Hedgehog (Autodesk Fusion 360 design; units mm, degrees)
Autodesk Fusion 360 part; units mm, degrees
note: some values were not read from the file. Set by a fixed rule: which sketch regions a step uses.
(part 1 of 2)
sketch "Sketch4" plane through (0, 0, 0) normal (0, 0, 1) x (1, 0, 0)
  line L0 (-34.7307, 191.5789) -> (1016.2208, 191.5789)
  line L1 (1016.2208, 191.5789) -> (1016.2208, -23.2363)
  line L2 (1016.2208, -23.2363) -> (-34.7307, -23.2363)
  line L3 (-34.7307, -23.2363) -> (-34.7307, 191.5789)
  line L4 (-14.0403, 161.1518) -> (163.6539, 161.1518)
  line L5 (163.6539, 161.1518) -> (163.6539, 10.2335)
  line L6 (163.6539, 10.2335) -> (-14.0403, 10.2335)
  line L7 (-14.0403, 10.2335) -> (-14.0403, 161.1518)
  spline S0 degree 3 poles (109.5886, 49.3104) (109.6257, 48.0501) (109.3099, 46.9639) (108.2091, 46.2939) knots 0 0 0 0 1 1 1 1
  spline S1 degree 3 poles (108.2091, 46.2939) (107.8993, 46.1052) (107.561, 45.9726) (107.2226, 45.8399) knots 0 0 0 0 1 1 1 1
  spline S2 degree 3 poles (107.2226, 45.8399) (106.9189, 45.7212) (106.6147, 45.602) (106.3317, 45.4419) knots 0 0 0 0 1 1 1 1
  spline S3 degree 3 poles (106.3317, 45.4419) (105.6678, 45.067) (105.1207, 44.4463) (104.9491, 43.7039) knots 0 0 0 0 1 1 1 1
  spline S4 degree 3 poles (104.9491, 43.7039) (104.7763, 42.9615) (105.0288, 42.1089) (105.6477, 41.6641) knots 0 0 0 0 1 1 1 1
  spline S5 degree 3 poles (105.6477, 41.6641) (106.1254, 41.3209) (106.7419, 41.2497) (107.3297, 41.215) knots 0 0 0 0 1 1 1 1
  spline S6 degree 3 poles (107.3297, 41.215) (111.923, 40.9454) (115.0552, 41.6239) (115.8079, 46.7503) knots 0 0 0 0 1 1 1 1
  spline S7 degree 3 poles (115.8079, 46.7503) (115.9868, 47.9716) (116.1183, 49.2307) (116.1183, 50.4764) knots 0 0 0 0 1 1 1 1
  spline S8 degree 3 poles (116.1183, 50.4764) (119.4056, 51.2164) (122.0869, 52.1176) (123.8121, 53.1838) knots 0 0 0 0 1 1 1 1
  spline S9 degree 3 poles (123.8121, 53.1838) (124.4796, 53.5958) (125.3535, 53.8209) (126.189, 54.0357) knots 0 0 0 0 1 1 1 1
  spline S10 degree 3 poles (126.189, 54.0357) (127.9082, 54.4781) (129.4685, 54.8798) (128.7577, 56.787) knots 0 0 0 0 1 1 1 1
  line L8 (128.7577, 56.787) -> (128.6384, 57.1442)
  spline S11 degree 3 poles (128.6384, 57.1442) (129.9656, 57.2215) (132.1333, 57.3943) (133.0443, 57.7314) knots 0 0 0 0 1 1 1 1
  spline S12 degree 2 poles (133.0443, 57.7314) (134.4098, 58.2371) (132.3493, 63.2089) knots 0 0 0 1 1 1
  spline S13 degree 2 poles (132.3493, 63.2089) (136.6432, 62.0015) (138.6368, 64.3663) knots 0 0 0 1 1 1
  spline S14 degree 2 poles (138.6368, 64.3663) (140.6522, 66.7567) (129.92, 74.047) knots 0 0 0 1 1 1
  spline S15 degree 2 poles (129.92, 74.047) (135.9093, 73.8967) (138.2637, 76.3917) knots 0 0 0 1 1 1
  spline S16 degree 2 poles (138.2637, 76.3917) (140.6474, 78.9184) (126.1945, 83.6042) knots 0 0 0 1 1 1
  spline S17 degree 2 poles (126.1945, 83.6042) (133.7788, 85.2917) (134.9922, 88.733) knots 0 0 0 1 1 1
  spline S18 degree 2 poles (134.9922, 88.733) (136.216, 92.2041) (121.0608, 94.2177) knots 0 0 0 1 1 1
  spline S19 degree 2 poles (121.0608, 94.2177) (130.8541, 97.9883) (130.6527, 101.1843) knots 0 0 0 1 1 1
  spline S20 degree 2 poles (130.6527, 101.1843) (130.4506, 104.3889) (113.1942, 101.9815) knots 0 0 0 1 1 1
  spline S21 degree 2 poles (113.1942, 101.9815) (122.5828, 107.2837) (121.0475, 109.7769) knots 0 0 0 1 1 1
  spline S22 degree 2 poles (121.0475, 109.7769) (119.5182, 112.2598) (100.8633, 108.6761) knots 0 0 0 1 1 1
  spline S23 degree 2 poles (100.8633, 108.6761) (113.2813, 116.3687) (110.9798, 119.6566) knots 0 0 0 1 1 1
  spline S24 degree 2 poles (110.9798, 119.6566) (107.9042, 124.0497) (89.2098, 113.5389) knots 0 0 0 1 1 1
  spline S25 degree 2 poles (89.2098, 113.5389) (99.8374, 122.5539) (97.3934, 126.0025) knots 0 0 0 1 1 1
  spline S26 degree 2 poles (97.3934, 126.0025) (94.9672, 129.4249) (77.9353, 116.7569) knots 0 0 0 1 1 1
  spline S27 degree 2 poles (77.9353, 116.7569) (83.1292, 123.5397) (81.9913, 126.8745) knots 0 0 0 1 1 1
  spline S28 degree 2 poles (81.9913, 126.8745) (80.8563, 130.2032) (63.1064, 114.8084) knots 0 0 0 1 1 1
  spline S29 degree 2 poles (63.1064, 114.8084) (68.0374, 122.6482) (66.5075, 124.7586) knots 0 0 0 1 1 1
  spline S30 degree 3 poles (66.5075, 124.7586) (65.3872, 126.3043) (56.8159, 118.2697) (51.9068, 113.6679) knots 0 0 0 0 1 1 1 1
  spline S31 degree 3 poles (51.9068, 113.6679) (50.1475, 112.0188) (48.8586, 110.8102) (48.5519, 110.6423) knots 0 0 0 0 1 1 1 1
  spline S32 degree 3 poles (48.5519, 110.6423) (48.1119, 110.4007) (48.3407, 111.3738) (48.6724, 112.788) knots 0 0 0 0 1 1 1 1
  spline S33 degree 3 poles (48.6724, 112.788) (49.2122, 115.0877) (50.0252, 118.5527) (48.6839, 119.8562) knots 0 0 0 0 1 1 1 1
  spline S34 degree 3 poles (48.6839, 119.8562) (46.9715, 121.5206) (41.6425, 110.8108) (38.6625, 104.821) knots 0 0 0 0 1 1 1 1
  spline S35 degree 3 poles (38.6625, 104.821) (37.9055, 103.2996) (37.3, 102.0831) (36.944, 101.4509) knots 0 0 0 0 1 1 1 1
  spline S36 degree 3 poles (36.944, 101.4509) (36.0518, 99.8662) (35.537, 101.7697) (34.8987, 104.1303) knots 0 0 0 0 1 1 1 1
  spline S37 degree 3 poles (34.8987, 104.1303) (34.2944, 106.3642) (33.5793, 109.0077) (32.3294, 109.494) knots 0 0 0 0 1 1 1 1
  spline S38 degree 3 poles (32.3294, 109.494) (29.7893, 110.4822) (30.3547, 93.6694) (30.6571, 90.6164) knots 0 0 0 0 1 1 1 1
  spline S39 degree 3 poles (30.6571, 90.6164) (30.8026, 89.1468) (29.053, 90.2245) (27.318, 91.2931) knots 0 0 0 0 1 1 1 1
  spline S40 degree 3 poles (27.318, 91.2931) (25.4549, 92.4402) (23.6081, 93.5776) (24.1413, 91.5414) knots 0 0 0 0 1 1 1 1
  spline S41 degree 2 poles (24.1413, 91.5414) (25.1718, 87.6041) (28.5546, 81.4019) knots 0 0 0 1 1 1
  spline S42 degree 2 poles (28.5546, 81.4019) (22.02, 79.7004) (25.3388, 77.663) knots 0 0 0 1 1 1
  spline S43 degree 3 poles (25.3388, 77.663) (27.4805, 76.3479) (29.9591, 72.7204) (31.4829, 70.2485) knots 0 0 0 0 1 1 1 1
  spline S44 degree 3 poles (31.4829, 70.2485) (24.6857, 66.904) (19.2909, 63.9525) (22.1953, 61.5847) knots 0 0 0 0 1 1 1 1
  spline S45 degree 3 poles (22.1953, 61.5847) (24.3014, 59.8674) (32.417, 58.4872) (39.0288, 57.3626) knots 0 0 0 0 1 1 1 1
  spline S46 degree 3 poles (39.0288, 57.3626) (41.7143, 56.9056) (44.1515, 56.4912) (45.8378, 56.1133) knots 0 0 0 0 1 1 1 1
  spline S47 degree 3 poles (45.8378, 56.1133) (47.005, 55.8522) (48.1685, 55.5248) (49.374, 55.1475) knots 0 0 0 0 1 1 1 1
  line L9 (49.374, 55.1475) -> (49.3771, 55.1342)
  spline S48 degree 3 poles (49.3771, 55.1342) (49.9089, 52.5886) (50.4609, 49.9488) (48.4138, 48.7718) knots 0 0 0 0 1 1 1 1
  spline S49 degree 3 poles (48.4138, 48.7718) (48.0998, 48.5911) (47.7584, 48.4676) (47.417, 48.3441) knots 0 0 0 0 1 1 1 1
  spline S50 degree 3 poles (47.417, 48.3441) (47.1096, 48.2321) (46.8023, 48.1207) (46.5145, 47.968) knots 0 0 0 0 1 1 1 1
  spline S51 degree 3 poles (46.5145, 47.968) (45.8421, 47.6101) (45.2792, 47.0034) (45.0887, 46.2659) knots 0 0 0 0 1 1 1 1
  spline S52 degree 3 poles (45.0887, 46.2659) (44.897, 45.5283) (45.1288, 44.6691) (45.7356, 44.209) knots 0 0 0 0 1 1 1 1
  spline S53 degree 3 poles (45.7356, 44.209) (46.2047, 43.8536) (46.8194, 43.7666) (47.406, 43.7173) knots 0 0 0 0 1 1 1 1
  spline S54 degree 3 poles (47.406, 43.7173) (51.9902, 43.3315) (55.1387, 43.9297) (56.0205, 49.036) knots 0 0 0 0 1 1 1 1
  spline S55 degree 3 poles (56.0205, 49.036) (56.2317, 50.2549) (56.3948, 51.5133) (56.4264, 52.7602) knots 0 0 0 0 1 1 1 1
  spline S56 degree 3 poles (56.4264, 52.7602) (57.8011, 52.2965) (59.2805, 51.814) (60.9004, 51.3241) knots 0 0 0 0 1 1 1 1
  spline S57 degree 3 poles (60.9004, 51.3241) (61.2741, 49.2471) (61.3453, 47.2943) (59.6645, 46.3279) knots 0 0 0 0 1 1 1 1
  spline S58 degree 3 poles (59.6645, 46.3279) (59.3505, 46.1478) (59.0097, 46.0243) (58.6683, 45.9001) knots 0 0 0 0 1 1 1 1
  spline S59 degree 3 poles (58.6683, 45.9001) (58.361, 45.7888) (58.0537, 45.6774) (57.7652, 45.5241) knots 0 0 0 0 1 1 1 1
  spline S60 degree 3 poles (57.7652, 45.5241) (57.0928, 45.1668) (56.5311, 44.5595) (56.3394, 43.822) knots 0 0 0 0 1 1 1 1
  spline S61 degree 3 poles (56.3394, 43.822) (56.1483, 43.0844) (56.379, 42.2258) (56.9863, 41.7657) knots 0 0 0 0 1 1 1 1
  spline S62 degree 3 poles (56.9863, 41.7657) (57.4549, 41.4097) (58.0701, 41.3227) (58.6567, 41.2734) knots 0 0 0 0 1 1 1 1
  spline S63 degree 3 poles (58.6567, 41.2734) (63.2415, 40.8876) (66.3895, 41.4864) (67.2719, 46.5921) knots 0 0 0 0 1 1 1 1
  spline S64 degree 3 poles (67.2719, 46.5921) (67.4368, 47.5432) (67.5719, 48.5187) (67.6382, 49.4942) knots 0 0 0 0 1 1 1 1
  spline S65 degree 3 poles (67.6382, 49.4942) (68.0222, 49.4011) (68.4129, 49.3086) (68.8109, 49.2167) knots 0 0 0 0 1 1 1 1
  spline S66 degree 3 poles (68.8109, 49.2167) (74.0942, 47.9929) (84.3688, 47.5682) (94.7646, 48.0142) knots 0 0 0 0 1 1 1 1
  spline S67 degree 3 poles (94.7646, 48.0142) (94.5473, 47.5968) (94.2205, 47.2359) (93.7519, 46.9505) knots 0 0 0 0 1 1 1 1
  spline S68 degree 3 poles (93.7519, 46.9505) (93.4422, 46.7624) (93.1044, 46.6298) (92.7667, 46.4977) knots 0 0 0 0 1 1 1 1
  spline S69 degree 3 poles (92.7667, 46.4977) (92.4624, 46.3785) (92.1576, 46.2592) (91.8734, 46.0985) knots 0 0 0 0 1 1 1 1
  spline S70 degree 3 poles (91.8734, 46.0985) (91.2101, 45.7243) (90.6636, 45.103) (90.492, 44.3605) knots 0 0 0 0 1 1 1 1
  spline S71 degree 3 poles (90.492, 44.3605) (90.3192, 43.6187) (90.5711, 42.7655) (91.1906, 42.3207) knots 0 0 0 0 1 1 1 1
  spline S72 degree 3 poles (91.1906, 42.3207) (91.6683, 41.9775) (92.2847, 41.9063) (92.872, 41.8722) knots 0 0 0 0 1 1 1 1
  spline S73 degree 3 poles (92.872, 41.8722) (97.4659, 41.602) (100.5968, 42.2799) (101.3496, 47.4063) knots 0 0 0 0 1 1 1 1
  spline S74 degree 3 poles (101.3496, 47.4063) (101.3995, 47.744) (101.4451, 48.0848) (101.4859, 48.4274) knots 0 0 0 0 1 1 1 1
  spline S75 degree 3 poles (101.4859, 48.4274) (104.2907, 48.6544) (107.0254, 48.9483) (109.5886, 49.3104) knots 0 0 0 0 1 1 1 1
  line L10 (193.4724, 161.1518) -> (371.1666, 161.1518)
  line L11 (371.1666, 161.1518) -> (371.1666, 10.2335)
  line L12 (371.1666, 10.2335) -> (193.4724, 10.2335)
  line L13 (193.4724, 10.2335) -> (193.4724, 161.1518)
  spline S76 degree 3 poles (261.6784, 59.7712) (261.0309, 60.2988) (260.2082, 60.5623) (259.3878, 60.7175) knots 0 0 0 0 1 1 1 1
  spline S77 degree 3 poles (259.3878, 60.7175) (257.7259, 61.0315) (256.9239, 60.5118) (256.5977, 59.5576) knots 0 0 0 0 1 1 1 1
  spline S78 degree 3 poles (256.5977, 59.5576) (255.6009, 56.6464) (259.3069, 50.7143) (255.9265, 48.7718) knots 0 0 0 0 1 1 1 1
  spline S79 degree 3 poles (255.9265, 48.7718) (255.3295, 48.4286) (254.6351, 48.2911) (254.0272, 47.968) knots 0 0 0 0 1 1 1 1
  spline S80 degree 3 poles (254.0272, 47.968) (253.3548, 47.6101) (252.7919, 47.0034) (252.6014, 46.2659) knots 0 0 0 0 1 1 1 1
  spline S81 degree 3 poles (252.6014, 46.2659) (252.4097, 45.5283) (252.6415, 44.6691) (253.2483, 44.209) knots 0 0 0 0 1 1 1 1
  spline S82 degree 3 poles (253.2483, 44.209) (253.7175, 43.8536) (254.3321, 43.7666) (254.9187, 43.7173) knots 0 0 0 0 1 1 1 1
  spline S83 degree 3 poles (254.9187, 43.7173) (259.5035, 43.3315) (262.6515, 43.9297) (263.5332, 49.036) knots 0 0 0 0 1 1 1 1
  spline S84 degree 3 poles (263.5332, 49.036) (264.0688, 52.1304) (264.297, 55.4768) (262.8413, 58.2596) knots 0 0 0 0 1 1 1 1
  spline S85 degree 3 poles (262.8413, 58.2596) (262.5444, 58.8268) (262.175, 59.3672) (261.6784, 59.7712) knots 0 0 0 0 1 1 1 1
  spline S86 degree 3 poles (306.736, 58.0917) (306.0764, 58.6022) (305.2463, 58.8456) (304.4224, 58.9795) knots 0 0 0 0 1 1 1 1
  spline S87 degree 3 poles (304.4224, 58.9795) (302.7544, 59.2509) (301.9651, 58.7124) (301.662, 57.7491) knots 0 0 0 0 1 1 1 1
  spline S88 degree 3 poles (301.662, 57.7491) (300.7407, 54.8147) (304.5952, 48.9781) (301.2647, 46.9505) knots 0 0 0 0 1 1 1 1
  spline S89 degree 3 poles (301.2647, 46.9505) (300.6762, 46.5927) (299.9861, 46.4369) (299.3861, 46.0985) knots 0 0 0 0 1 1 1 1
  spline S90 degree 3 poles (299.3861, 46.0985) (298.7228, 45.7243) (298.1763, 45.103) (298.0047, 44.3605) knots 0 0 0 0 1 1 1 1
  spline S91 degree 3 poles (298.0047, 44.3605) (297.8319, 43.6187) (298.0838, 42.7655) (298.7033, 42.3207) knots 0 0 0 0 1 1 1 1
  spline S92 degree 3 poles (298.7033, 42.3207) (299.181, 41.9775) (299.7975, 41.9063) (300.3853, 41.8722) knots 0 0 0 0 1 1 1 1
  spline S93 degree 3 poles (300.3853, 41.8722) (304.9786, 41.602) (308.1095, 42.2799) (308.8623, 47.4063) knots 0 0 0 0 1 1 1 1
  spline S94 degree 3 poles (308.8623, 47.4063) (309.3193, 50.5141) (309.4629, 53.8641) (307.9367, 56.6099) knots 0 0 0 0 1 1 1 1
  spline S95 degree 3 poles (307.9367, 56.6099) (307.6257, 57.1691) (307.243, 57.7004) (306.736, 58.0917) knots 0 0 0 0 1 1 1 1
  line L14 (335.9661, 57.6998) -> (335.3576, 58.3083)
  spline S96 degree 2 poles (335.3576, 58.3083) (334.174, 58.4331) (333.5362, 58.8603) knots 0 0 0 1 1 1
  spline S97 degree 3 poles (333.5362, 58.8603) (332.8972, 59.2868) (332.271, 59.7901) (331.5152, 59.9252) knots 0 0 0 0 1 1 1 1
  spline S98 degree 3 poles (331.5152, 59.9252) (331.6211, 58.7678) (331.8493, 57.6213) (332.1956, 56.5101) knots 0 0 0 0 1 1 1 1
  spline S99 degree 3 poles (332.1956, 56.5101) (329.9391, 56.6938) (328.1494, 58.4306) (326.6725, 60.1467) knots 0 0 0 0 1 1 1 1
  spline S100 degree 3 poles (326.6725, 60.1467) (326.1789, 60.7206) (325.5966, 61.4441) (324.8493, 61.4539) knots 0 0 0 0 1 1 1 1
  spline S101 degree 3 poles (324.8493, 61.4539) (324.7878, 60.9536) (327.6151, 55.4159) (326.4552, 55.6752) knots 0 0 0 0 1 1 1 1
  spline S102 degree 2 poles (326.4552, 55.6752) (324.7866, 56.0488) (313.0271, 62.1853) knots 0 0 0 1 1 1
  spline S103 degree 2 poles (313.0271, 62.1853) (315.7571, 54.0437) (313.4969, 54.8999) knots 0 0 0 1 1 1
  spline S104 degree 2 poles (313.4969, 54.8999) (311.2368, 55.7567) (302.27, 63.8071) knots 0 0 0 1 1 1
  spline S105 degree 2 poles (302.27, 63.8071) (301.9608, 56.1711) (300.238, 57.0815) knots 0 0 0 1 1 1
  spline S106 degree 2 poles (300.238, 57.0815) (298.5159, 57.9925) (289.95, 67.4419) knots 0 0 0 1 1 1
  spline S107 degree 2 poles (289.95, 67.4419) (289.2392, 58.4075) (286.3603, 60.0153) knots 0 0 0 1 1 1
  spline S108 degree 2 poles (286.3603, 60.0153) (283.4806, 61.6236) (276.9004, 72.9042) knots 0 0 0 1 1 1
  spline S109 degree 2 poles (276.9004, 72.9042) (282.7412, 84.9058) (273.8699, 84.0034) knots 0 0 0 1 1 1
  spline S110 degree 3 poles (273.8699, 84.0034) (269.7592, 83.5847) (266.3277, 82.0366) (264.4211, 78.1614) knots 0 0 0 0 1 1 1 1
  spline S111 degree 3 poles (264.4211, 78.1614) (262.9338, 79.7558) (260.6427, 80.4464) (258.4671, 80.3083) knots 0 0 0 0 1 1 1 1
  spline S112 degree 3 poles (258.4671, 80.3083) (256.4151, 80.099) (255.0283, 79.547) (253.1631, 78.6391) knots 0 0 0 0 1 1 1 1
  spline S113 degree 3 poles (253.1631, 78.6391) (252.7274, 78.4273) (252.2204, 78.2125) (251.7774, 78.4078) knots 0 0 0 0 1 1 1 1
  spline S114 degree 3 poles (251.7774, 78.4078) (251.4865, 78.5356) (251.2961, 78.8119) (251.0959, 79.0578) knots 0 0 0 0 1 1 1 1
  spline S115 degree 3 poles (251.0959, 79.0578) (250.3413, 79.987) (249.2343, 80.64) (248.0458, 80.7781) knots 0 0 0 0 1 1 1 1
  spline S116 degree 3 poles (248.0458, 80.7781) (246.8446, 80.9175) (244.5838, 80.3253) (244.2108, 78.9379) knots 0 0 0 0 1 1 1 1
  spline S117 degree 3 poles (244.2108, 78.9379) (244.6575, 80.5998) (245.3025, 82.9658) (244.5966, 84.6551) knots 0 0 0 0 1 1 1 1
  spline S118 degree 3 poles (244.5966, 84.6551) (244.4676, 84.9643) (244.2498, 85.2375) (243.979, 85.459) knots 0 0 0 0 1 1 1 1
  spline S119 degree 3 poles (243.979, 85.459) (243.1246, 86.16) (241.7407, 86.3505) (240.9442, 85.5472) knots 0 0 0 0 1 1 1 1
  spline S120 degree 3 poles (240.9442, 85.5472) (240.3161, 84.9138) (240.2875, 83.8768) (240.5839, 83.0352) knots 0 0 0 0 1 1 1 1
  spline S121 degree 3 poles (240.5839, 83.0352) (240.8803, 82.1942) (241.442, 81.4773) (241.8972, 80.7099) knots 0 0 0 0 1 1 1 1
  spline S122 degree 3 poles (241.8972, 80.7099) (242.8781, 79.0529) (243.7581, 76.4678) (243.1714, 74.557) knots 0 0 0 0 1 1 1 1
  spline S123 degree 3 poles (243.1714, 74.557) (242.628, 72.7886) (241.0141, 71.2392) (239.3985, 70.4469) knots 0 0 0 0 1 1 1 1
  spline S124 degree 3 poles (239.3985, 70.4469) (232.4142, 67.0202) (226.7463, 63.9994) (229.7081, 61.5847) knots 0 0 0 0 1 1 1 1
  spline S125 degree 3 poles (229.7081, 61.5847) (232.6698, 59.17) (247.514, 57.4217) (253.3505, 56.1133) knots 0 0 0 0 1 1 1 1
  spline S126 degree 3 poles (253.3505, 56.1133) (259.187, 54.8061) (264.9183, 51.8584) (276.3236, 49.2167) knots 0 0 0 0 1 1 1 1
  spline S127 degree 3 poles (276.3236, 49.2167) (287.7276, 46.575) (322.3817, 47.6564) (331.3248, 53.1838) knots 0 0 0 0 1 1 1 1
  spline S128 degree 3 poles (331.3248, 53.1838) (333.3658, 54.4435) (337.3268, 53.9518) (336.2704, 56.787) knots 0 0 0 0 1 1 1 1
  line L15 (336.2704, 56.787) -> (335.9661, 57.6998)
  spline S129 degree 3 poles (272.9291, 57.328) (272.2816, 57.8549) (271.4589, 58.1184) (270.6386, 58.2736) knots 0 0 0 0 1 1 1 1
  spline S130 degree 3 poles (270.6386, 58.2736) (268.9779, 58.5876) (268.1752, 58.0691) (267.8484, 57.1137) knots 0 0 0 0 1 1 1 1
  spline S131 degree 3 poles (267.8484, 57.1137) (266.8522, 54.2037) (270.5576, 48.2716) (267.1772, 46.3279) knots 0 0 0 0 1 1 1 1
  spline S132 degree 3 poles (267.1772, 46.3279) (266.5802, 45.986) (265.8865, 45.8472) (265.2779, 45.5241) knots 0 0 0 0 1 1 1 1
  spline S133 degree 3 poles (265.2779, 45.5241) (264.6055, 45.1668) (264.0438, 44.5595) (263.8521, 43.822) knots 0 0 0 0 1 1 1 1
  spline S134 degree 3 poles (263.8521, 43.822) (263.661, 43.0844) (263.8917, 42.2258) (264.499, 41.7657) knots 0 0 0 0 1 1 1 1
  spline S135 degree 3 poles (264.499, 41.7657) (264.9676, 41.4097) (265.5828, 41.3227) (266.1694, 41.2734) knots 0 0 0 0 1 1 1 1
  spline S136 degree 3 poles (266.1694, 41.2734) (270.7542, 40.8876) (273.9022, 41.4864) (274.7846, 46.5921) knots 0 0 0 0 1 1 1 1
  spline S137 degree 3 poles (274.7846, 46.5921) (275.3195, 49.6871) (275.5483, 53.0329) (274.092, 55.8157) knots 0 0 0 0 1 1 1 1
  spline S138 degree 3 poles (274.092, 55.8157) (273.7951, 56.3829) (273.4257, 56.9239) (272.9291, 57.328) knots 0 0 0 0 1 1 1 1
  spline S139 degree 3 poles (321.1938, 57.4351) (320.5335, 57.9456) (319.7041, 58.1884) (318.8807, 58.3229) knots 0 0 0 0 1 1 1 1
  spline S140 degree 3 poles (318.8807, 58.3229) (317.2115, 58.5949) (316.4222, 58.0558) (316.1204, 57.0931) knots 0 0 0 0 1 1 1 1
  spline S141 degree 3 poles (316.1204, 57.0931) (315.1978, 54.158) (319.0523, 48.3215) (315.7218, 46.2939) knots 0 0 0 0 1 1 1 1
  spline S142 degree 3 poles (315.7218, 46.2939) (315.1345, 45.9361) (314.4432, 45.7797) (313.8444, 45.4419) knots 0 0 0 0 1 1 1 1
  spline S143 degree 3 poles (313.8444, 45.4419) (313.1805, 45.067) (312.6334, 44.4463) (312.4618, 43.7039) knots 0 0 0 0 1 1 1 1
  spline S144 degree 3 poles (312.4618, 43.7039) (312.289, 42.9615) (312.5415, 42.1089) (313.1604, 41.6641) knots 0 0 0 0 1 1 1 1
  spline S145 degree 3 poles (313.1604, 41.6641) (313.6381, 41.3209) (314.2546, 41.2497) (314.8424, 41.215) knots 0 0 0 0 1 1 1 1
  spline S146 degree 3 poles (314.8424, 41.215) (319.4357, 40.9454) (322.5678, 41.6239) (323.3206, 46.7503) knots 0 0 0 0 1 1 1 1
  spline S147 degree 3 poles (323.3206, 46.7503) (323.7764, 49.8575) (323.9201, 53.2081) (322.3944, 55.9526) knots 0 0 0 0 1 1 1 1
  spline S148 degree 3 poles (322.3944, 55.9526) (322.0828, 56.5125) (321.7001, 57.0444) (321.1938, 57.4351) knots 0 0 0 0 1 1 1 1
  line L16 (400.9851, 161.1518) -> (578.6793, 161.1518)
  line L17 (578.6793, 161.1518) -> (578.6793, 10.2335)
  line L18 (578.6793, 10.2335) -> (400.9851, 10.2335)
  line L19 (400.9851, 10.2335) -> (400.9851, 161.1518)
  spline S149 degree 3 poles (454.1419, 80.6777) (454.6585, 80.7909) (455.1655, 80.8237) (455.5586, 80.7781) knots 0 0 0 0 1 1 1 1
  spline S150 degree 3 poles (455.5586, 80.7781) (456.7471, 80.64) (457.854, 79.987) (458.6086, 79.0578) knots 0 0 0 0 1 1 1 1
  spline S151 degree 3 poles (458.6086, 79.0578) (458.6353, 79.0249) (458.6621, 78.9908) (458.6895, 78.9567) knots 0 0 0 0 1 1 1 1
  spline S152 degree 3 poles (458.6895, 78.9567) (458.8623, 78.7401) (459.0388, 78.518) (459.2901, 78.4078) knots 0 0 0 0 1 1 1 1
  spline S153 degree 3 poles (459.2901, 78.4078) (459.7332, 78.2125) (460.2401, 78.4273) (460.6758, 78.6391) knots 0 0 0 0 1 1 1 1
  spline S154 degree 3 poles (460.6758, 78.6391) (462.541, 79.547) (463.9278, 80.099) (465.9798, 80.3083) knots 0 0 0 0 1 1 1 1
  spline S155 degree 3 poles (465.9798, 80.3083) (468.1554, 80.4464) (470.4465, 79.7558) (471.9338, 78.1614) knots 0 0 0 0 1 1 1 1
  spline S156 degree 3 poles (471.9338, 78.1614) (473.8404, 82.0366) (477.2719, 83.5847) (481.3826, 84.0034) knots 0 0 0 0 1 1 1 1
  spline S157 degree 3 poles (481.3826, 84.0034) (488.9712, 84.775) (485.7946, 76.1063) (484.7174, 73.5821) knots 0 0 0 0 1 1 1 1
  spline S158 degree 3 poles (484.7174, 73.5821) (485.5809, 73.3009) (486.4098, 72.8871) (487.1887, 72.4173) knots 0 0 0 0 1 1 1 1
  spline S159 degree 3 poles (487.1887, 72.4173) (486.8321, 73.3874) (486.6654, 74.4268) (486.7019, 75.4594) knots 0 0 0 0 1 1 1 1
  spline S160 degree 3 poles (486.7019, 75.4594) (486.9629, 75.3487) (487.224, 75.2379) (487.4851, 75.1278) knots 0 0 0 0 1 1 1 1
  spline S161 degree 3 poles (487.4851, 75.1278) (487.8575, 74.9702) (488.2299, 74.8126) (488.6024, 74.6543) knots 0 0 0 0 1 1 1 1
  spline S162 degree 3 poles (488.6024, 74.6543) (488.603, 76.3303) (488.603, 78.005) (488.603, 79.6803) knots 0 0 0 0 1 1 1 1
  spline S163 degree 3 poles (488.603, 79.6803) (489.3697, 79.101) (490.2941, 78.7316) (491.2495, 78.6239) knots 0 0 0 0 1 1 1 1
  spline S164 degree 3 poles (491.2495, 78.6239) (490.3519, 80.304) (489.8067, 82.1723) (489.66, 84.0715) knots 0 0 0 0 1 1 1 1
  spline S165 degree 3 poles (489.66, 84.0715) (492.5348, 82.6725) (495.533, 81.5284) (498.6086, 80.6582) knots 0 0 0 0 1 1 1 1
  spline S166 degree 3 poles (498.6086, 80.6582) (495.8531, 84.7087) (492.6571, 88.4597) (489.0971, 91.825) knots 0 0 0 0 1 1 1 1
  spline S167 degree 3 poles (489.0971, 91.825) (493.6027, 91.7982) (498.106, 91.3984) (502.5459, 90.6322) knots 0 0 0 0 1 1 1 1
  spline S168 degree 3 poles (502.5459, 90.6322) (496.842, 95.1452) (489.3588, 97.3456) (482.119, 96.6373) knots 0 0 0 0 1 1 1 1
  spline S169 degree 3 poles (482.119, 96.6373) (484.2178, 97.4893) (486.2911, 98.4069) (488.3328, 99.3897) knots 0 0 0 0 1 1 1 1
  spline S170 degree 3 poles (488.3328, 99.3897) (480.9792, 101.4083) (472.6202, 99.2102) (467.2109, 93.8368) knots 0 0 0 0 1 1 1 1
  spline S171 degree 3 poles (467.2109, 93.8368) (467.5742, 96.3245) (468.4815, 98.7307) (469.8496, 100.8405) knots 0 0 0 0 1 1 1 1
  spline S172 degree 3 poles (469.8496, 100.8405) (464.2473, 98.5621) (459.6188, 93.9883) (457.2734, 88.4135) knots 0 0 0 0 1 1 1 1
  line L20 (457.2734, 88.4135) -> (457.5558, 95.2036)
  spline S173 degree 3 poles (457.5558, 95.2036) (454.3755, 91.2201) (453.9782, 85.8783) (454.1419, 80.6777) knots 0 0 0 0 1 1 1 1
  line L21 (608.4979, 161.1518) -> (786.192, 161.1518)
  line L22 (786.192, 161.1518) -> (786.192, 10.2335)
  line L23 (786.192, 10.2335) -> (608.4979, 10.2335)
  line L24 (608.4979, 10.2335) -> (608.4979, 161.1518)
  spline S174 degree 3 poles (656.0676, 85.6379) (656.8769, 86.3347) (658.1853, 86.1327) (659.0068, 85.459) knots 0 0 0 0 1 1 1 1
  spline S175 degree 3 poles (659.0068, 85.459) (659.2745, 85.2375) (659.4937, 84.9643) (659.6214, 84.6551) knots 0 0 0 0 1 1 1 1
  spline S176 degree 3 poles (659.6214, 84.6551) (660.3213, 82.9786) (659.6945, 80.6363) (659.2442, 78.9762) knots 0 0 0 0 1 1 1 1
  line L25 (659.2442, 78.9762) -> (659.2381, 78.9379)
  spline S177 degree 3 poles (659.2381, 78.9379) (659.6093, 80.3253) (661.873, 80.9175) (663.0719, 80.7781) knots 0 0 0 0 1 1 1 1
  spline S178 degree 3 poles (663.0719, 80.7781) (664.2585, 80.64) (665.366, 79.987) (666.1206, 79.0578) knots 0 0 0 0 1 1 1 1
  spline S179 degree 3 poles (666.1206, 79.0578) (666.1511, 79.0249) (666.1755, 78.9908) (666.1997, 78.9567) knots 0 0 0 0 1 1 1 1
  spline S180 degree 3 poles (666.1997, 78.9567) (666.3762, 78.7401) (666.5527, 78.518) (666.8023, 78.4078) knots 0 0 0 0 1 1 1 1
  spline S181 degree 3 poles (666.8023, 78.4078) (667.2465, 78.2125) (667.7516, 78.4273) (668.1897, 78.6391) knots 0 0 0 0 1 1 1 1
  spline S182 degree 3 poles (668.1897, 78.6391) (670.0519, 79.547) (671.4394, 80.099) (673.4901, 80.3083) knots 0 0 0 0 1 1 1 1
  spline S183 degree 3 poles (673.4901, 80.3083) (675.6687, 80.4464) (677.9568, 79.7558) (679.4477, 78.1614) knots 0 0 0 0 1 1 1 1
  spline S184 degree 3 poles (679.4477, 78.1614) (681.3524, 82.0366) (684.7846, 83.5847) (688.8923, 84.0034) knots 0 0 0 0 1 1 1 1
  spline S185 degree 3 poles (688.8923, 84.0034) (697.2658, 84.8541) (692.5435, 74.2259) (691.9776, 73.0162) knots 0 0 0 0 1 1 1 1
  spline S186 degree 3 poles (691.9776, 73.0162) (692.4766, 72.8184) (692.9574, 72.5774) (693.4199, 72.2883) knots 0 0 0 0 1 1 1 1
  spline S187 degree 3 poles (693.4199, 72.2883) (693.645, 72.1453) (693.8702, 71.9895) (694.1075, 71.8319) knots 0 0 0 0 1 1 1 1
  spline S188 degree 3 poles (694.1075, 71.8319) (695.2272, 71.0688) (696.4078, 70.2643) (697.637, 70.6867) knots 0 0 0 0 1 1 1 1
  spline S189 degree 3 poles (697.637, 70.6867) (697.9657, 71.6615) (698.2943, 72.6364) (698.6168, 73.6113) knots 0 0 0 0 1 1 1 1
  spline S190 degree 3 poles (698.6168, 73.6113) (698.702, 73.8572) (698.7811, 74.103) (698.8663, 74.3489) knots 0 0 0 0 1 1 1 1
  spline S191 degree 3 poles (698.8663, 74.3489) (702.0307, 71.9256) (705.2012, 69.5024) (708.3656, 67.0786) knots 0 0 0 0 1 1 1 1
  spline S192 degree 3 poles (708.3656, 67.0786) (708.2621, 68.2939) (708.1648, 69.5091) (708.0614, 70.7238) knots 0 0 0 0 1 1 1 1
  spline S193 degree 3 poles (708.0614, 70.7238) (707.9519, 72.0413) (707.8423, 73.3582) (707.7327, 74.675) knots 0 0 0 0 1 1 1 1
  spline S194 degree 3 poles (707.7327, 74.675) (711.5909, 71.2915) (715.6803, 68.1667) (719.9523, 65.3303) knots 0 0 0 0 1 1 1 1
  spline S195 degree 3 poles (719.9523, 65.3303) (719.9948, 66.2978) (720.0375, 67.2654) (720.074, 68.233) knots 0 0 0 0 1 1 1 1
  spline S196 degree 3 poles (720.074, 68.233) (720.1166, 69.2061) (720.1592, 70.1791) (720.1957, 71.1528) knots 0 0 0 0 1 1 1 1
  spline S197 degree 3 poles (720.1957, 71.1528) (723.8226, 68.4411) (727.4434, 65.7307) (731.0703, 63.0202) knots 0 0 0 0 1 1 1 1
  line L26 (731.0703, 63.0202) -> (731.1007, 62.9971)
  spline S198 degree 3 poles (731.1007, 62.9971) (730.7295, 65.1002) (730.5957, 67.2466) (730.7052, 69.3795) knots 0 0 0 0 1 1 1 1
  spline S199 degree 3 poles (730.7052, 69.3795) (733.2794, 67.2021) (736.2612, 65.5086) (739.4439, 64.4132) knots 0 0 0 0 1 1 1 1
  spline S200 degree 3 poles (739.4439, 64.4132) (739.024, 67.8874) (738.1963, 71.3122) (736.9975, 74.5996) knots 0 0 0 0 1 1 1 1
  spline S201 degree 3 poles (736.9975, 74.5996) (739.383, 73.1318) (741.811, 71.7382) (744.2818, 70.4213) knots 0 0 0 0 1 1 1 1
  spline S202 degree 3 poles (744.2818, 70.4213) (744.0931, 74.0896) (742.4926, 77.6666) (739.882, 80.2541) knots 0 0 0 0 1 1 1 1
  spline S203 degree 3 poles (739.882, 80.2541) (739.5047, 80.6296) (739.097, 80.9984) (738.6892, 81.3696) knots 0 0 0 0 1 1 1 1
  spline S204 degree 3 poles (738.6892, 81.3696) (737.0706, 82.8447) (735.4032, 84.3575) (735.2571, 86.4698) knots 0 0 0 0 1 1 1 1
  line L27 (735.2571, 86.4698) -> (742.1944, 85.7907)
  spline S205 degree 3 poles (742.1944, 85.7907) (739.3587, 89.4236) (735.1719, 91.9795) (730.6443, 92.8467) knots 0 0 0 0 1 1 1 1
  spline S206 degree 3 poles (730.6443, 92.8467) (729.8594, 92.9958) (728.8248, 93.4412) (729.0257, 94.2117) knots 0 0 0 0 1 1 1 1
  spline S207 degree 3 poles (729.0257, 94.2117) (729.1838, 94.7843) (729.9263, 94.9176) (730.5166, 94.9297) knots 0 0 0 0 1 1 1 1
  spline S208 degree 3 poles (730.5166, 94.9297) (732.9751, 94.9815) (735.4396, 94.8616) (737.886, 94.5701) knots 0 0 0 0 1 1 1 1
  spline S209 degree 3 poles (737.886, 94.5701) (735.8108, 97.182) (732.3908, 98.3382) (729.0804, 98.7636) knots 0 0 0 0 1 1 1 1
  spline S210 degree 3 poles (729.0804, 98.7636) (727.6443, 98.9485) (726.1898, 99.021) (724.7415, 99.0934) knots 0 0 0 0 1 1 1 1
  spline S211 degree 3 poles (724.7415, 99.0934) (722.855, 99.1871) (720.9746, 99.2808) (719.1186, 99.621) knots 0 0 0 0 1 1 1 1
  spline S212 degree 3 poles (719.1186, 99.621) (718.7778, 100.5752) (720.0861, 101.2342) (721.0842, 101.3766) knots 0 0 0 0 1 1 1 1
  spline S213 degree 3 poles (721.0842, 101.3766) (723.7557, 101.7564) (726.4697, 101.8531) (729.1656, 101.6651) knots 0 0 0 0 1 1 1 1
  spline S214 degree 3 poles (729.1656, 101.6651) (729.4333, 102.8128) (728.6666, 104.0055) (727.6503, 104.6007) knots 0 0 0 0 1 1 1 1
  spline S215 degree 3 poles (727.6503, 104.6007) (726.6341, 105.1952) (725.417, 105.3242) (724.2364, 105.4167) knots 0 0 0 0 1 1 1 1
  spline S216 degree 3 poles (724.2364, 105.4167) (720.2808, 105.7283) (716.301, 105.7813) (712.3333, 105.5725) knots 0 0 0 0 1 1 1 1
  spline S217 degree 3 poles (712.3333, 105.5725) (712.5159, 107.0774) (714.3415, 107.6556) (715.8203, 108.0036) knots 0 0 0 0 1 1 1 1
  spline S218 degree 3 poles (715.8203, 108.0036) (717.299, 108.3505) (719.0881, 109.2938) (718.8508, 110.7914) knots 0 0 0 0 1 1 1 1
  spline S219 degree 3 poles (718.8508, 110.7914) (711.9438, 110.7476) (705.0491, 109.7307) (698.4282, 107.7821) knots 0 0 0 0 1 1 1 1
  spline S220 degree 3 poles (698.4282, 107.7821) (697.8561, 108.8459) (698.8419, 110.0636) (699.7791, 110.8273) knots 0 0 0 0 1 1 1 1
  spline S221 degree 3 poles (699.7791, 110.8273) (700.7224, 111.5898) (701.8116, 112.6383) (701.4526, 113.7927) knots 0 0 0 0 1 1 1 1
  spline S222 degree 3 poles (701.4526, 113.7927) (697.9596, 114.3063) (694.43, 113.155) (691.2473, 111.636) knots 0 0 0 0 1 1 1 1
  spline S223 degree 3 poles (691.2473, 111.636) (690.158, 111.1163) (689.0871, 110.5516) (688.016, 109.9875) knots 0 0 0 0 1 1 1 1
  spline S224 degree 3 poles (688.016, 109.9875) (685.9592, 108.9012) (683.9084, 107.8156) (681.7115, 107.0549) knots 0 0 0 0 1 1 1 1
  spline S225 degree 3 poles (681.7115, 107.0549) (681.8941, 108.729) (682.3931, 110.3678) (683.172, 111.8618) knots 0 0 0 0 1 1 1 1
  spline S226 degree 3 poles (683.172, 111.8618) (679.3564, 110.8127) (675.9364, 108.3968) (673.6666, 105.1545) knots 0 0 0 0 1 1 1 1
  spline S227 degree 3 poles (673.6666, 105.1545) (672.7659, 103.8662) (671.3115, 102.2408) (669.9727, 103.0684) knots 0 0 0 0 1 1 1 1
  line L28 (669.9727, 103.0684) -> (671.2202, 108.3529)
  spline S228 degree 3 poles (671.2202, 108.3529) (670.1796, 108.6079) (669.2546, 107.6811) (668.6035, 106.8316) knots 0 0 0 0 1 1 1 1
  spline S229 degree 3 poles (668.6035, 106.8316) (665.9442, 103.3599) (663.6622, 99.6045) (661.7939, 95.6503) knots 0 0 0 0 1 1 1 1
  spline S230 degree 3 poles (661.7939, 95.6503) (660.9237, 95.3314) (660.1265, 96.3324) (659.9196, 97.2385) knots 0 0 0 0 1 1 1 1
  spline S231 degree 3 poles (659.9196, 97.2385) (659.8771, 97.4357) (659.8405, 97.6396) (659.804, 97.844) knots 0 0 0 0 1 1 1 1
  spline S232 degree 3 poles (659.804, 97.844) (659.6762, 98.5822) (659.5423, 99.3325) (658.9825, 99.8029) knots 0 0 0 0 1 1 1 1
  spline S233 degree 3 poles (658.9825, 99.8029) (657.4003, 96.0622) (656.3597, 92.0915) (655.9033, 88.0538) knots 0 0 0 0 1 1 1 1
  line L29 (655.9033, 88.0538) -> (655.9033, 86.9098)
  spline S234 degree 2 poles (655.9033, 86.9098) (655.8667, 86.5915) (656.0676, 85.6379) knots 0 0 0 1 1 1
  line L30 (816.0106, 161.1518) -> (993.7047, 161.1518)
  line L31 (993.7047, 161.1518) -> (993.7047, 10.2335)
  line L32 (993.7047, 10.2335) -> (816.0106, 10.2335)
  line L33 (816.0106, 10.2335) -> (816.0106, 161.1518)
  spline S235 degree 3 poles (854.586, 65.9145) (853.6306, 66.1287) (852.6326, 66.1317) (851.6894, 65.8585) knots 0 0 0 0 1 1 1 1
  spline S236 degree 3 poles (851.6894, 65.8585) (850.7766, 65.5932) (849.8516, 65.0674) (850.1436, 64.0365) knots 0 0 0 0 1 1 1 1
  spline S237 degree 3 poles (850.1436, 64.0365) (850.6853, 62.1342) (852.091, 60.594) (853.6793, 60.2313) knots 0 0 0 0 1 1 1 1
  spline S238 degree 3 poles (853.6793, 60.2313) (855.2615, 59.8692) (857.2514, 62.9326) (856.9411, 64.3992) knots 0 0 0 0 1 1 1 1
  spline S239 degree 3 poles (856.9411, 64.3992) (856.7585, 65.2536) (855.5719, 65.6942) (854.586, 65.9145) knots 0 0 0 0 1 1 1 1
  spline S240 degree 3 poles (897.7438, 82.2386) (895.9486, 82.4072) (894.0865, 82.1534) (892.4981, 81.3106) knots 0 0 0 0 1 1 1 1
  spline S241 degree 3 poles (892.4981, 81.3106) (890.9098, 80.4671) (889.6137, 79.0012) (889.1755, 77.2552) knots 0 0 0 0 1 1 1 1
  spline S242 degree 3 poles (889.1755, 77.2552) (889.0417, 76.7356) (889.0477, 76.0655) (889.5163, 75.8051) knots 0 0 0 0 1 1 1 1
  spline S243 degree 3 poles (889.5163, 75.8051) (889.7841, 75.6584) (890.1066, 75.701) (890.4109, 75.7491) knots 0 0 0 0 1 1 1 1
  spline S244 degree 3 poles (890.4109, 75.7491) (892.8511, 76.1368) (893.7457, 75.9834) (894.5368, 73.5492) knots 0 0 0 0 1 1 1 1
  spline S245 degree 3 poles (894.5368, 73.5492) (894.8472, 72.5999) (897.9264, 76.0558) (898.0481, 76.3625) knots 0 0 0 0 1 1 1 1
  spline S246 degree 3 poles (898.0481, 76.3625) (898.4862, 77.4804) (898.4984, 78.7194) (898.4132, 79.9188) knots 0 0 0 0 1 1 1 1
  spline S247 degree 3 poles (898.4132, 79.9188) (898.3584, 80.7343) (898.2489, 81.5954) (897.7438, 82.2386) knots 0 0 0 0 1 1 1 1
  spline S248 degree 3 poles (877.1082, 75.0189) (875.7632, 75.2787) (874.4184, 74.1553) (874.0958, 72.5098) knots 0 0 0 0 1 1 1 1
  spline S249 degree 3 poles (874.0958, 72.5098) (873.7795, 70.8643) (874.6132, 69.3199) (875.9519, 69.06) knots 0 0 0 0 1 1 1 1
  spline S250 degree 3 poles (875.9519, 69.06) (877.2968, 68.7996) (878.6417, 69.9235) (878.9642, 71.569) knots 0 0 0 0 1 1 1 1
  spline S251 degree 3 poles (878.9642, 71.569) (879.2806, 73.2145) (878.453, 74.7584) (877.1082, 75.0189) knots 0 0 0 0 1 1 1 1
  spline S252 degree 3 poles (868.4547, 76.026) (867.2924, 76.2512) (866.124, 75.2769) (865.8441, 73.8499) knots 0 0 0 0 1 1 1 1
  spline S253 degree 3 poles (865.8441, 73.8499) (865.5702, 72.4216) (866.2883, 71.0822) (867.4567, 70.8564) knots 0 0 0 0 1 1 1 1
  spline S254 degree 3 poles (867.4567, 70.8564) (868.619, 70.6307) (869.7874, 71.6056) (870.0673, 73.0326) knots 0 0 0 0 1 1 1 1
  spline S255 degree 3 poles (870.0673, 73.0326) (870.3412, 74.4596) (869.6231, 75.8002) (868.4547, 76.026) knots 0 0 0 0 1 1 1 1
extrude "Extrude6" add sketch "Sketch4" along normal blind 2 contours S0 S1 S2 S3 S4 S5 S6 S7 S8 S9 S10 L8 S11 S12 S13 S14 S15 S16 S17 S18 S19 S20 S21 S22 S23 S24 S25 S26 S27 S28 S29 S30 S31 S32 S33 S34 S35 S36 S37 S38 S39 S40 S41 S42 S43 S44 S45 S46 S47 L9 S48 S49 S50 S51 S52 S53 S54 S55 S56 S57 S58 S59 S60 S61 S62 S63 S64 S65 S66 S67 S68 S69 S70 S71 S72 S73 S74 S75 makes body 1
extrude "Extrude7" add sketch "Sketch4" along normal blind 4 separate body contours S76 S77 S78 S84 S85 S126 | S76 S77 S78 S84 S85 S86 S87 S88 S94 S95 L14 S96 S97 S98 S99 S100 S101 S102 S103 S104 S105 S106 S107 S108 S109 S110 S111 S112 S113 S114 S115 S116 S117 S118 S119 S120 S121 S122 S123 S124 S125 S126 S127 S128 L15 S129 S130 S131 S137 S138 S139 S140 S141 S147 S148 | S78 S79 S80 S81 S82 S83 S84 S126 | S126 S129 S130 S131 S137 S138 | S126 S131 S132 S133 S134 S135 S136 S137 | S88 S89 S90 S91 S92 S93 S94 S127 | S86 S87 S88 S94 S95 S127 | S127 S139 S140 S141 S147 S148 | S127 S141 S142 S143 S144 S145 S146 S147 makes body 2
extrude "Extrude8" add sketch "Sketch4" along normal blind 2 separate body contours S149 S150 S151 S152 S153 S154 S155 S156 S157 S158 S159 S160 S161 S162 S163 S164 S165 S166 S167 S168 S169 S170 S171 S172 L20 S173 makes body 3
extrude "Extrude10" add sketch "Sketch4" along normal blind 2 separate body contours S235 S236 S237 S238 S239 | S240 S241 S242 S243 S244 S245 S246 S247 | S248 S249 S250 S251 | S252 S253 S254 S255 makes body 4 at (895.0782, 78.7656, 0) makes body 5 at (877.3757, 72.1126, 0) makes body 6 at (854.1668, 62.9487, 0) makes body 7 at (867.222, 73.3774, 0)